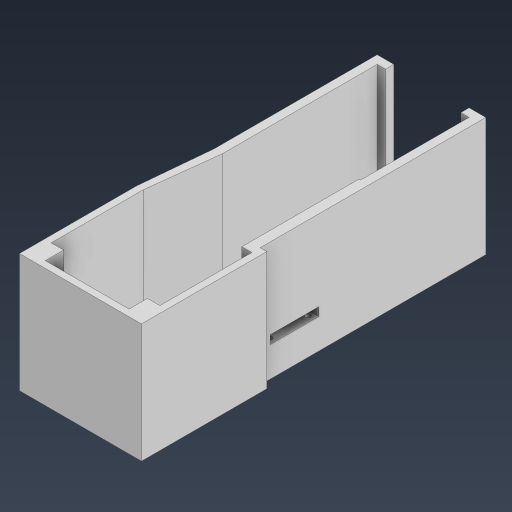
# Autodesk Inventor part: New_base
Saved by Autodesk Inventor 2024 (Build 280153000, 153)
## iProperties
Created: 2025-10-20
Part Number: New_base
Material: Generic
Document SubType Name: Modeling
Designer: Piter
Density: 1 g/cm^3
Appearance: Default
Author: Piter
Autodesk Inventor part; units mm, degrees
ref_plane "YZ Plane" through (0, 0, 0) normal (1, 0, 0) x (0, 1, 0)
ref_plane "XZ Plane" through (0, 0, 0) normal (0, 1, 0) x (-1, 0, 0)
ref_plane "XY Plane" through (0, 0, 0) normal (0, 0, 1) x (1, 0, 0)
sketch "Sketch1" plane through (0, 0, 0) normal (0, 1, 0) x (-1, 0, 0)
  line L0 (-22.5, 32.5) -> (22.5, 32.5) construction
  line L1 (22.5, 32.5) -> (22.5, -32.5) construction
  line L2 (22.5, -32.5) -> (-22.5, -32.5) construction
  line L3 (-22.5, -32.5) -> (-22.5, 32.5) construction
  line L4 (-22.5, 32.5) -> (22.5, -32.5) construction
  line L5 (22.5, 32.5) -> (-22.5, -32.5) construction
  circle A0 centre (22.5, 32.5) radius 1.5
  circle A1 centre (22.5, -32.5) radius 1.5
  circle A2 centre (-22.5, -32.5) radius 1.5
  circle A3 centre (-22.5, 32.5) radius 1.5
  line L6 (27.5, 30) -> (-27.5, 30)
  line L7 (-27.5, 30) -> (-27.5, 37.5)
  line L8 (-27.5, 37.5) -> (27.5, 37.5)
  line L9 (27.5, 37.5) -> (27.5, 30)
  line L10 (27.5, -30) -> (27.5, -37.5)
  line L11 (27.5, -37.5) -> (-27.5, -37.5)
  line L12 (-27.5, -37.5) -> (-27.5, -30)
  line L13 (-27.5, -30) -> (27.5, -30)
  circle A4 centre (22.5, 32.5) radius 5
  circle A5 centre (22.5, -32.5) radius 5
  circle A6 centre (-22.5, -32.5) radius 5
  circle A7 centre (-22.5, 32.5) radius 5
  line L14 (-27.5, 37.5) -> (27.5, 37.5)
  line L15 (27.5, 37.5) -> (27.5, -37.5)
  line L16 (27.5, -37.5) -> (-27.5, -37.5)
  line L17 (-27.5, -37.5) -> (-27.5, 37.5)
  line L18 (-27.5, 37.5) -> (27.5, -37.5) construction
  line L19 (27.5, 37.5) -> (-27.5, -37.5) construction
  line L20 (-32.5, 42.5) -> (32.5, 42.5)
  line L21 (32.5, 42.5) -> (32.5, -42.5)
  line L22 (32.5, -42.5) -> (-32.5, -42.5)
  line L23 (-32.5, -42.5) -> (-32.5, 42.5)
  line L24 (-32.5, 42.5) -> (32.5, -42.5) construction
  line L25 (32.5, 42.5) -> (-32.5, -42.5) construction
  line L26 (32.5, 42.5) -> (-14.872, 42.5)
  line L27 (0, 0) -> (0, -184) construction
  line L28 (-22.5, -47.5) -> (22.5, -47.5)
  line L29 (22.5, -47.5) -> (22.5, -92.5)
  line L30 (22.5, -92.5) -> (-22.5, -92.5)
  line L31 (-22.5, -92.5) -> (-22.5, -47.5)
  line L32 (-22.5, -47.5) -> (22.5, -92.5) construction
  line L33 (22.5, -47.5) -> (-22.5, -92.5) construction
  line L34 (32.5, -42.5) -> (32.5, -97.5)
  line L35 (32.5, -97.5) -> (-32.5, -97.5)
  line L36 (-32.5, -97.5) -> (-32.5, -42.5)
  line L37 (22.5, 27.5) -> (27.5, 27.5)
  line L38 (22.5, -27.5) -> (27.5, -27.5)
  line L39 (-22.5, -27.5) -> (-27.5, -27.5)
  line L40 (-22.5, 27.5) -> (-27.5, 27.5)
  line L41 (0, 0) -> (0, 113) construction
  line L42 (32.5, 42.5) -> (32.5, 97.5)
  line L43 (32.5, 97.5) -> (-32.5, 97.5)
  line L44 (-32.5, 97.5) -> (-32.5, 42.5)
  line L45 (29.5, 42.5) -> (29.5, 97.5)
  line L46 (-29.5, 97.5) -> (-29.5, 42.5)
  line L47 (32.5, 42.5) -> (36.5, 42.5)
  line L48 (36.5, 42.5) -> (36.5, 112.5)
  line L49 (36.5, 112.5) -> (-36.5, 112.5)
  line L50 (-36.5, 112.5) -> (-36.5, 42.5)
  line L51 (-36.5, 42.5) -> (-32.5, 42.5)
  line L52 (36.5, 42.5) -> (32.5, 0)
  line L53 (-27.5, 37.5) -> (-36.5, 37.5)
  line L54 (-36.5, 37.5) -> (-36.5, 42.5)
  line L55 (-27.5, -27.5) -> (-26.5, -27.5)
  line L56 (-26.5, -27.5) -> (-26.5, 27.5)
  point P0 (0, -70)
  point P1 (18.1699, 30)
  point P2 (18.1699, -30)
  point P3 (-18.1699, -30)
  point P4 (-18.1699, 30)
  point P5 (-32.5, 70)
  point P6 (-32.5, 37.5)
  dimension "d8" = 10
  dimension "d9" = 10
  dimension "d10" = 10
  dimension "d11" = 10
  dimension "d0" = 45
  dimension "d1" = 65
  dimension "d2" = 3
  dimension "d3" = 3
  dimension "d4" = 3
  dimension "d5" = 3
  dimension "d6" = 2.5
  dimension "d7" = 2.5
  dimension "d12" = 5
  dimension "d13" = 5
  dimension "d17" = 45
  dimension "d18" = 45
  dimension "d19" = 5
  dimension "d20" = 5
  dimension "d38" = 55
  dimension "d39" = 3
  dimension "d40" = 3
  dimension "d41" = 4
  dimension "d42" = 4
  dimension "d43" = 15
  dimension "d57" = 1
  constraints: 115 end point, 25 perpendicular, 18 point on line, 13 horizontal, 10 midpoint, 8 coincident, 8 parallel, 8 vertical, 4 centre point, 12 other
  measures "d0" distance of L1.end L2.end
  measures "d1" distance of L0.end L1.end
  measures "d2" diameter of A0
  measures "d3" diameter of A1
  measures "d4" diameter of A2
  measures "d5" diameter of A3
  measures "d6" distance from line of A0.centre L6
  measures "d7" distance from line of L1.end L13
  measures "d12" distance between parallel lines of L15 L21
  measures "d13" distance between parallel lines of L22 L16
  measures "d17" distance of L29.end L30.end
  measures "d18" distance of L28.end L29.end
  measures "d19" distance between parallel lines of L22 L28
  measures "d20" distance between parallel lines of L30 L35
  measures "d38" distance of L20.end L42.end
  measures "d39" distance from line of point (-32.5, 70) L46
  measures "d40" distance between parallel lines of L42 L45
  measures "d41" distance between parallel lines of L50 L44
  measures "d42" distance between parallel lines of L48 L42
  measures "d43" distance between parallel lines of L49 L43
  measures "d57" distance of L39.end L55.end
extrude "Extrusion1" add sketch "Sketch1" along normal blind 6 contours L15 L37 A4 L6 | L6 A4 L9 | A4 L6 | L6 A4 | A4 L8 L9 | L6 A7 L8 A4 | L15 L13 A5 L38 | A7 L6 | L6 A7 | A7 L7 L8 | L10 A5 L13 | A5 L13 | A7 L40 L17 L6 | L6 L7 A7 | A5 L13 | L10 L11 A5 | A5 L11 A6 L13 | A6 L13 | L13 A6 | L39 A6 L13 L17 | L11 L12 A6 | A6 L12 L13 | L44 L43 L46 L20 | L20 L21 L22 L23 | L51 L50 L49 L48 L47 L42 L43 L44 | L23 L53 L54 L51 | L22 L34 L35 L36 | L45 L43 L42 L20 | L47 L52 L21
sketch "Sketch3" plane through (0, 6, 0) normal (0, 1, 0) x (1, 0, 0)
  line L0 (29.5, -42.5) -> (29.5, -97.5) projected
  line L1 (29.5, -97.5) -> (-29.5, -97.5) projected
  line L2 (-29.5, -97.5) -> (-29.5, -42.5) projected
  line L3 (-29.5, -42.5) -> (29.5, -42.5) projected
  circle A0 centre (-22.5, -32.5) radius 1.5 projected
  circle A1 centre (22.5, 32.5) radius 1.5 projected
  line L4 (22.5, 47.5) -> (-22.5, 47.5) projected
  line L5 (-22.5, 47.5) -> (-22.5, 92.5) projected
  line L6 (-22.5, 92.5) -> (22.5, 92.5) projected
  line L7 (22.5, 92.5) -> (22.5, 47.5) projected
  circle A2 centre (22.5, -32.5) radius 1.5 projected
  circle A3 centre (-22.5, 32.5) radius 1.5 projected
  arc A4 (-18.1699, -30) -> (-22.5, -27.5) centre (-22.5, -32.5) ccw projected
  line L8 (-22.5, -27.5) -> (-27.5, -27.5) projected
  line L9 (-27.5, -27.5) -> (-27.5, 27.5) projected
  line L10 (-27.5, 27.5) -> (-22.5, 27.5) projected
  arc A5 (-22.5, 27.5) -> (-18.1699, 30) centre (-22.5, 32.5) ccw projected
  line L11 (-18.1699, 30) -> (18.1699, 30) projected
  arc A6 (18.1699, 30) -> (22.5, 27.5) centre (22.5, 32.5) ccw projected
  line L12 (22.5, 27.5) -> (27.5, 27.5) projected
  line L13 (27.5, 27.5) -> (27.5, -27.5) projected
  line L14 (27.5, -27.5) -> (22.5, -27.5) projected
  arc A7 (22.5, -27.5) -> (18.1699, -30) centre (22.5, -32.5) ccw projected
  line L15 (18.1699, -30) -> (-18.1699, -30) projected
  line L16 (32.5, -37.5) -> (32.5, 97.5) projected
  line L17 (32.5, 97.5) -> (-32.5, 97.5) projected
  line L18 (-32.5, 97.5) -> (-32.5, 0) projected
  line L19 (-32.5, 0) -> (-36.5, -42.5) projected
  line L20 (-36.5, -42.5) -> (-36.5, -112.5) projected
  line L21 (-36.5, -112.5) -> (36.5, -112.5) projected
  line L22 (-29.5, -97.5) -> (-32.5, -97.5)
  line L23 (-29.5, -97.5) -> (-29.5, -42.5) projected
  line L24 (-29.5, -42.5) -> (-32.5, -42.5)
  line L25 (-32.5, -42.5) -> (-32.5, -97.5)
  line L26 (29.5, -97.5) -> (32.5, -97.5)
  line L27 (32.5, -97.5) -> (32.5, -42.5)
  line L28 (32.5, -42.5) -> (29.5, -42.5)
  line L29 (-32.5, 0) -> (-27.5, 0)
  line L30 (-32.5, -42.5) -> (-27.5, 0)
  line L31 (-27.5, 27.5) -> (-27.5, 97.5)
  line L32 (27.5, 27.5) -> (27.5, 97.5)
  line L33 (-22.5, 92.5) -> (-22.5, 97.5)
  line L34 (32.5, 97.5) -> (-32.5, 97.5) projected
  line L35 (22.5, 92.5) -> (27.5, 92.5)
  line L36 (22.5, 92.5) -> (22.5, 97.5)
  line L37 (-22.5, 92.5) -> (-27.5, 92.5)
  line L38 (36.5, -112.5) -> (36.5, -37.5) projected
  line L39 (36.5, -37.5) -> (32.5, -37.5) projected
  line L40 (27.5, -27.5) -> (27.5, -42.5)
  line L41 (32.5, -31.5) -> (27.5, -31.5)
  line L42 (32.5, -2.5) -> (27.5, -2.5)
  line L43 (27.5, -31.5) -> (27.5, -2.5)
  line L44 (27.5, -17) -> (32.5, -17) construction
  point P0 (0, 0)
  point P1 (27.5, 0)
  point P2 (30, -2.5)
  point P3 (30, -31.5)
  dimension "d44" = 3
  dimension "d45" = 3
  dimension "d48" = 29
  dimension "d49" = 1
  constraints: 38 end point, 14 point on line, 10 perpendicular, 5 midpoint, 4 horizontal, 1 collinear
  measures "d44" distance between parallel lines of L2 L25
  measures "d45" distance of L0.end L26.end
  measures "d48" distance from line of L41 point (30, -2.5)
  measures "d49" vertical distance of A2.centre point (30, -31.5)
extrude "Extrusion3" add sketch "Sketch3" along normal blind 15 contours L3 L40 L41 L16 L39 L38 L21 L20 L19 L29 L30 L25 L22 L1 L26 L27 L28 | L29 L18 L17 L31 L9 | L13 L32 L17 L16 L42 | L31 L17 L33 L37 | L35 L36 L17 L32
sketch "Sketch4" plane through (0, 6, 0) normal (0, 1, 0) x (1, 0, 0)
  line L0 (-32.5, 0) -> (-36.5, -42.5) projected
  line L1 (-36.5, -42.5) -> (-36.5, -112.5) projected
  line L2 (-36.5, -112.5) -> (36.5, -112.5) projected
  line L3 (36.5, -112.5) -> (36.5, -37.5) projected
  line L4 (36.5, -37.5) -> (32.5, -37.5) projected
  line L5 (32.5, -37.5) -> (32.5, -31.5) projected
  line L6 (32.5, -31.5) -> (27.5, -31.5) projected
  line L7 (27.5, -31.5) -> (27.5, -42.5) projected
  line L8 (27.5, -42.5) -> (32.5, -42.5) projected
  line L9 (32.5, -42.5) -> (32.5, -97.5) projected
  line L10 (32.5, -97.5) -> (-32.5, -97.5) projected
  line L11 (-32.5, -97.5) -> (-32.5, -42.5) projected
  line L12 (-32.5, -42.5) -> (-27.5, 0) projected
  line L13 (-27.5, 0) -> (-27.5, 92.5) projected
  line L14 (-27.5, 92.5) -> (-22.5, 92.5) projected
  line L15 (-22.5, 92.5) -> (-22.5, 97.5) projected
  line L16 (-22.5, 97.5) -> (-32.5, 97.5) projected
  line L17 (-32.5, 97.5) -> (-32.5, 0) projected
  line L18 (32.5, -2.5) -> (27.5, -2.5) projected
  line L19 (27.5, -2.5) -> (27.5, -27.5) projected
  line L20 (27.5, -27.5) -> (22.5, -27.5) projected
  arc A0 (22.5, -27.5) -> (18.1699, -30) centre (22.5, -32.5) ccw projected
  line L21 (18.1699, -30) -> (-18.1699, -30) projected
  arc A1 (-18.1699, -30) -> (-22.5, -27.5) centre (-22.5, -32.5) ccw projected
  line L22 (-22.5, -27.5) -> (-27.5, -27.5) projected
  line L23 (-27.5, -27.5) -> (-27.5, 0) projected
  line L24 (-27.5, 0) -> (-32.5, -42.5) projected
  line L25 (-32.5, -42.5) -> (-32.5, -97.5) projected
  line L26 (-32.5, -97.5) -> (-29.5, -97.5) projected
  line L27 (-29.5, -97.5) -> (-29.5, -42.5) projected
  line L28 (-29.5, -42.5) -> (27.5, -42.5) projected
  line L29 (27.5, -42.5) -> (27.5, -31.5) projected
  line L30 (27.5, -31.5) -> (32.5, -31.5) projected
  line L31 (32.5, -31.5) -> (32.5, -2.5) projected
  circle A2 centre (-22.5, -32.5) radius 1.5 projected
  circle A3 centre (22.5, -32.5) radius 1.5 projected
  line L32 (32.5, -2.5) -> (32.5, 97.5) projected
  line L33 (27.5, -31.5) -> (27.5, -27.5)
  circle A4 centre (29, -28.5) radius 1.5
  circle A5 centre (29, -5.5) radius 1.5
  line L34 (29, -28.5) -> (29, -3.5194)
  line L35 (27.5, 92.5) -> (22.5, 92.5) projected
  line L36 (22.5, 92.5) -> (22.5, 47.5) projected
  line L37 (22.5, 47.5) -> (-22.5, 47.5) projected
  line L38 (-22.5, 47.5) -> (-22.5, 92.5) projected
  line L39 (-22.5, 92.5) -> (-27.5, 92.5) projected
  line L40 (-27.5, 92.5) -> (-27.5, 27.5) projected
  line L41 (-27.5, 27.5) -> (-22.5, 27.5) projected
  arc A6 (-22.5, 27.5) -> (-18.1699, 30) centre (-22.5, 32.5) ccw projected
  line L42 (-18.1699, 30) -> (18.1699, 30) projected
  arc A7 (18.1699, 30) -> (22.5, 27.5) centre (22.5, 32.5) ccw projected
  line L43 (22.5, 27.5) -> (27.5, 27.5) projected
  line L44 (27.5, 27.5) -> (27.5, 92.5) projected
  circle A8 centre (22.5, 32.5) radius 1.5 projected
  circle A9 centre (-22.5, 32.5) radius 1.5 projected
  line L45 (32.5, -2.5) -> (32.5, 97.5) projected
  line L46 (32.5, 97.5) -> (22.5, 97.5) projected
  line L47 (22.5, 97.5) -> (22.5, 92.5) projected
  line L48 (22.5, 92.5) -> (27.5, 92.5) projected
  line L49 (27.5, 92.5) -> (27.5, -2.5) projected
  line L50 (27.5, -2.5) -> (32.5, -2.5) projected
  line L51 (26.5, -27.5) -> (26.5, 27.5)
  line L52 (26.5, -27.5) -> (26.5, -42.5)
  line L53 (27.5, -31.5) -> (26.5, -31.5)
  line L54 (27.5, -2.5) -> (26.5, -2.5)
  line L55 (26.5, 27.5) -> (26.5, 92.5)
  point P0 (0, 0)
  point P1 (27.5, -5.5)
  point P2 (27.5, -28.5)
  dimension "d52" = 3
  dimension "d53" = 3
  dimension "d54" = 6.5
  dimension "d55" = 4
  dimension "d56" = 23
  dimension "d58" = 1
  constraints: 14 end point, 7 point on line, 5 perpendicular, 2 centre point, 1 collinear, 1 vertical
  measures "d52" diameter of A4
  measures "d53" diameter of A5
  measures "d54" horizontal distance of L34.start A0.centre
  measures "d55" vertical distance of A0.centre L34.start
  measures "d56" distance of A5.centre L34.start
  measures "d58" distance between parallel lines of L49 L51
extrude "Extrusion4" add sketch "Sketch4" along normal blind 12 contours L6 L33 A4 L34 A5 L19 L18 L31 | L53 L52 L20 L33 | L7 L28 L52 L53 | L35 L44 L43 L55 | L33 L19 A5 L34 A4 | L54 L51 L43 L49 | L19 L20 L51 L54
extrude "Extrusion5" add sketch "Sketch4" against normal up to surface (6 mm away) contours L54 L51 L43 L49 | L19 L20 L51 L54
extrude "Extrusion6" add sketch "Sketch4" along normal up to surface (15 mm away) contours L7 L28 L52 L53 | L54 L51 L43 L49
sketch "Sketch5" plane through (0, 21, 0) normal (0, 1, 0) x (1, 0, 0)
  line L0 (-32.5, 0) -> (-36.5, -42.5) projected
  line L1 (-36.5, -42.5) -> (-36.5, -112.5) projected
  line L2 (-36.5, -112.5) -> (36.5, -112.5) projected
  line L3 (36.5, -112.5) -> (36.5, -37.5) projected
  line L4 (36.5, -37.5) -> (32.5, -37.5) projected
  line L5 (32.5, -37.5) -> (32.5, -31.5) projected
  line L6 (32.5, -31.5) -> (26.5, -31.5) projected
  line L7 (26.5, -42.5) -> (26.5, -31.5) projected
  line L8 (32.5, -42.5) -> (26.5, -42.5) projected
  line L9 (32.5, -42.5) -> (32.5, -97.5) projected
  line L10 (32.5, -97.5) -> (-32.5, -97.5) projected
  line L11 (-32.5, -97.5) -> (-32.5, -42.5) projected
  line L12 (-32.5, -42.5) -> (-27.5, 0) projected
  line L13 (-27.5, 0) -> (-27.5, 92.5) projected
  line L14 (-27.5, 92.5) -> (-22.5, 92.5) projected
  line L15 (-22.5, 92.5) -> (-22.5, 97.5) projected
  line L16 (-22.5, 97.5) -> (-32.5, 97.5) projected
  line L17 (-32.5, 97.5) -> (-32.5, 0) projected
  line L18 (0, -97.5) -> (0, -112.5)
  line L19 (25.05, -112.5) -> (-25.05, -112.5)
  line L20 (-25.05, -112.5) -> (-25.05, -97.5)
  line L21 (-25.05, -97.5) -> (25.05, -97.5)
  line L22 (25.05, -97.5) -> (25.05, -112.5)
  line L23 (25.05, -112.5) -> (-25.05, -97.5) construction
  line L24 (-25.05, -112.5) -> (25.05, -97.5) construction
  line L25 (-25.05, -108.5) -> (25.05, -108.5)
  circle A0 centre (29, -28.5) radius 1.5 projected
  circle A1 centre (29, -5.5) radius 1.5 projected
  line L26 (26.5, -2.5) -> (32.5, -2.5) projected
  line L27 (26.5, -2.5) -> (26.5, -31.5) projected
  line L28 (26.5, -31.5) -> (32.5, -31.5) projected
  line L29 (32.5, -31.5) -> (32.5, -2.5) projected
  line L30 (32.5, -2.5) -> (32.5, 97.5) projected
  line L31 (32.5, -2.5) -> (32.5, 97.5) projected
  line L32 (32.5, 97.5) -> (22.5, 97.5) projected
  line L33 (22.5, 97.5) -> (22.5, 92.5) projected
  line L34 (22.5, 92.5) -> (27.5, 92.5) projected
  line L35 (27.5, 92.5) -> (27.5, 27.5) projected
  line L36 (26.5, 27.5) -> (27.5, 27.5) projected
  line L37 (26.5, -2.5) -> (26.5, 27.5) projected
  line L38 (32.5, -2.5) -> (26.5, -2.5) projected
  point P0 (0, 0)
  point P1 (0, -105)
  dimension "d63" = 50.1
  dimension "d64" = 4
  constraints: 16 end point, 5 midpoint, 3 point on line, 2 parallel, 2 perpendicular, 1 horizontal
  measures "d63" distance of L20.end L21.end
  measures "d64" distance between parallel lines of L2 L25
extrude "Extrusion7" add sketch "Sketch5" along normal blind 50.1 contours L17 L16 L15 L14 L13 L12 L11 L10 L20 L2 L1 L0 | L20 L25 L18 L2 | L18 L25 L22 L2 | L22 L10 L9 L8 L7 L6 L5 L4 L3 L2
move faces "Move1" translate (0, 2, 0) faces at (30.8333, 21, -40.8333)
sketch "Sketch6" plane through (22.5, 23, -97.5) normal (0, 1, 0) x (1, 0, 0)
  circle A0 centre (6.5, -126) radius 1.5 projected
  circle A1 centre (6.5, -103) radius 1.5 projected
  line L0 (4, -100) -> (10, -100) projected
  line L1 (4, -100) -> (4, -129) projected
  line L2 (4, -129) -> (10, -129) projected
  line L3 (10, -129) -> (10, -100) projected
  line L4 (10, -100) -> (10, 0) projected
  line L5 (10, 0) -> (0, 0) projected
  line L6 (0, 0) -> (0, -5) projected
  line L7 (0, -5) -> (5, -5) projected
  line L8 (5, -5) -> (5, -70) projected
  line L9 (4, -70) -> (5, -70) projected
  line L10 (4, -100) -> (4, -70) projected
  line L11 (10, -100) -> (4, -100) projected
  point P0 (-22.5, -97.5)
extrude "Extrusion8" add sketch "Sketch6" along normal up to surface (48.1 mm away) contours A0 | A1 | L10 L9 L8 L7 L6 L5 L4 L0 | L0 L3 L2 L1
body "Solid1"
